Autodesk Fusion 360 part; units mm, degrees
(part 2 of 2)
  constraint tangent L247 A253
  constraint tangent L251 A253
  constraint concentric A111 A254
  constraint concentric A112 A255
  constraint tangent L109 A256
  constraint tangent L109 A257
  constraint tangent A258 L252
  constraint tangent L108 A259
  constraint tangent L252 A259
  constraint tangent L108 A260
  constraint tangent L199 A261
  constraint tangent L200 A261
  constraint tangent L192 A262
  constraint tangent L193 A262
  constraint tangent L174 A263
  constraint tangent L190 A263
  constraint tangent L183 A264
  constraint tangent L184 A264
  measures "d1" diameter of A0
  measures "d2" diameter of A1
  measures "d3" diameter of A2
  measures "d4" diameter of A3
  measures "d5" diameter of A4
  measures "d9" diameter of A111
  measures "d12" diameter of A112
  measures "d305" diameter of A254
  measures "d306" diameter of A255
extrude "Extrude1" add sketch "mriya-bumper-sla" along normal blind 10.5 contours L106 L107 L211 A215 L212 L228 L229 A231 | L106 L107 L202 A206 L203 A207 L204 A208 L205 A209 L206 A210 L207 A211 L208 A212 L209 A213 L210 A214 L211 L212 A216 L213 A217 L214 A218 L215 A219 L216 A220 L217 A221 L218 A222 L219 A223 L220 A224 L221 A225 L222 A226 L223 A227 L224 L225 L226 L227 L228 L229 L230 L231 L232 L233 L234 L235 L236 L237 L238 L239 L240 L241 L242 L243 L244 L245 A228 A229 A230 A232 A233 A234 A235 A236 A237 A238 A239 A240 A241 A242 A243 A244 A245 A246 A247 A248 A249 makes body 1
extrude "Extrude2" add sketch "mriya-bumper-sla" along normal blind 17 contours L106 L107 L211 A215 L212 L228 L229 A231 bodies 1
extrude "Extrude3" add sketch "mriya-bumper-sla" along normal blind 2 from surface at 1.7 contours L108 L109 L202 A206 L203 A207 L204 A208 L205 A209 L206 A210 L207 A211 L208 A212 L209 A213 L210 A214 L211 L212 A216 L213 A217 L214 A218 L215 A219 L216 A220 L217 A221 L218 A222 L219 A223 L220 A224 L221 A225 L222 A226 L223 A227 A256 A257 A258 L252 A259 A260 | L109 L212 A256 A257 | L108 L211 A215 L212 A258 L252 A259 A260 | A114 | A115 | A116 | A117 | A254 | A255 bodies 1
extrude "Extrude6" add sketch "mriya-bumper-sla" along normal blind 1 from surface at 14.3 contours L108 L211 A215 L212 A258 L252 A259 A260 bodies 1
extrude "Extrude14" add sketch "mriya-bumper-sla" along normal blind 1 from surface at 7.7 contours L109 L212 A256 A257 bodies 1
chamfer "Chamfer5" distance 0.599 angle 45 4 edges at (-14.85, 78.0932, 14.3) (-7.4686, 77.6246, 14.3) (-7, 58.2443, 14.3) (-7, 9.5932, 7.7) on bodies 1
sketch "power-switch" plane through (-4.5, 0, 0) normal (1, 0, 0) x (0, 1, 0)
  line L0 (1.9932, 0) -> (76.4932, 0)
  line L1 (76.4932, 0) -> (76.4932, 17)
  line L2 (76.4932, 17) -> (19.2932, 17)
  line L3 (19.2932, 17) -> (19.2932, 10.5)
  line L4 (19.2932, 10.5) -> (1.9932, 10.5)
  line L5 (1.9932, 10.5) -> (1.9932, 0)
  line L6 (36.0432, 5.4) -> (25.7432, 5.4)
  line L7 (25.7432, 5.4) -> (25.7432, 8.2)
  line L8 (25.7432, 8.2) -> (36.0432, 8.2)
  line L9 (36.0432, 8.2) -> (36.0432, 5.4)
  line L10 (36.6432, 3.8) -> (25.1432, 3.8)
  line L11 (24.1432, 4.8) -> (24.1432, 8.8)
  line L12 (25.1432, 9.8) -> (36.6432, 9.8)
  line L13 (37.6432, 8.8) -> (37.6432, 4.8)
  arc A0 (25.1432, 9.8) -> (24.1432, 8.8) centre (25.1432, 8.8) ccw
  arc A1 (37.6432, 8.8) -> (36.6432, 9.8) centre (36.6432, 8.8) ccw
  arc A2 (36.6432, 3.8) -> (37.6432, 4.8) centre (36.6432, 4.8) ccw
  arc A3 (24.1432, 4.8) -> (25.1432, 3.8) centre (25.1432, 4.8) ccw
  line L14 (19.2932, 10.5) -> (1.8932, 10.5)
  line L15 (1.8932, 10.5) -> (1.8932, 0)
  line L16 (1.8932, 0) -> (76.5932, 0)
  line L17 (76.5932, 0) -> (76.5932, 17)
  line L18 (76.5932, 17) -> (19.2932, 17)
  line L19 (19.2932, 17) -> (19.2932, 10.5)
  constraint perpendicular L6 L7
  constraint tangent L11 A0
  constraint tangent L12 A0
  constraint tangent L12 A1
  constraint tangent L13 A1
  constraint tangent L10 A2
  constraint tangent L13 A2
  constraint tangent L10 A3
  constraint tangent L11 A3
  constraint vertical L7
  constraint perpendicular L7 L8
  constraint vertical L9
extrude "Extrude8" cut sketch "power-switch" against normal blind 2.5 contours L6 L7 L8 L9 bodies 1
extrude "Extrude9" cut sketch "power-switch" against normal blind 1 contours L10 L11 L12 L13 A0 A1 A2 A3 bodies 1
chamfer "Chamfer4" distance 0.5 angle 45 4 edges at (-7, 30.8932, 5.4) (-7, 36.0432, 6.8) (-7, 30.8932, 8.2) (-7, 25.7432, 6.8) on bodies 1
sketch "usb-c" plane through (0, 80.5932, 0) normal (0, 1, 0) x (-1, 0, 0)
  line L0 (8.5, 0) -> (41.1088, 0)
  line L1 (41.1088, 0) -> (41.1088, 10.5)
  line L2 (41.1088, 10.5) -> (25.8, 10.5)
  line L3 (25.8, 10.5) -> (25.8, 17)
  line L4 (25.8, 17) -> (8.5, 17)
  line L5 (8.5, 17) -> (8.5, 0)
  line L6 (10.9002, 11.05) -> (10.9002, 10.15)
  arc A0 (21.0002, 11.05) -> (19.7002, 12.35) centre (19.7002, 11.05) ccw
  arc A1 (11.8003, 10.15) -> (13.1003, 8.85) centre (13.1002, 10.15) ccw
  line L7 (21.9002, 11.05) -> (21.9002, 10.15)
  line L8 (13.1002, 12.35) -> (19.7002, 12.35)
  line L9 (11.8003, 10.15) -> (11.8003, 11.05)
  line L10 (13.1002, 13.25) -> (19.7002, 13.25)
  line L11 (19.7002, 7.95) -> (13.1002, 7.95)
  arc A2 (13.1002, 12.35) -> (11.8003, 11.05) centre (13.1002, 11.05) ccw
  line L12 (19.7002, 8.85) -> (13.1002, 8.85)
  line L13 (21.0002, 11.05) -> (21.0002, 10.15)
  arc A3 (19.7002, 8.85) -> (21.0002, 10.15) centre (19.7003, 10.15) ccw
  arc A4 (13.1002, 13.25) -> (10.9002, 11.05) centre (13.1002, 11.05) ccw
  arc A5 (10.9002, 10.15) -> (13.1002, 7.95) centre (13.1002, 10.15) ccw
  arc A6 (21.9002, 11.05) -> (19.7003, 13.25) centre (19.7003, 11.05) ccw
  arc A7 (19.7002, 7.95) -> (21.9002, 10.15) centre (19.7002, 10.15) ccw
  constraint horizontal L11
  constraint tangent L9 A2
  constraint tangent L8 A2
  constraint tangent A1 L12
  constraint tangent A1 L9
  constraint tangent A0 L8
  constraint tangent A0 L13
  constraint tangent L13 A3
  constraint tangent L12 A3
  constraint parallel L7 L9
  constraint tangent L6 A4
  constraint tangent L10 A4
  constraint tangent L11 A5
  constraint tangent L6 A5
  constraint tangent L10 A6
  constraint tangent L7 A6
  constraint tangent L7 A7
  constraint tangent L11 A7
extrude "Extrude10" cut sketch "usb-c" against normal blind 2.5 contours A0 A1 L8 L9 A2 L12 L13 A3 bodies 1
extrude "Extrude11" cut sketch "usb-c" against normal blind 1 contours L6 L7 L10 L11 A4 A5 A6 A7 bodies 1
fillet "Fillet30" radius 0.5 4 edges at (-5.75, 19.2932, 10.5) (-5.75, 19.2932, 17) (-25.8, 79.3432, 10.5) (-25.8, 79.3432, 17) on bodies 1
fillet "Fillet27" radius 1.2 90 edges at (-4.5, 47.9432, 17) (-5.6716, 79.4216, 17) (-17.15, 80.5932, 17) (-33.4544, 80.5932, 10.5) (-41.4915, 80.6693, 10.5) (-42.3069, 81.3771, 10.5) (-43.9334, 82.6268, 10.5) (-51.5908, 82.8932, 10.5) (-58.2915, 82.9693, 10.5) (-60.2069, 84.7771, 10.5) (-62.9334, 87.1268, 10.5) (-73.4, 87.3932, 10.5) (-83.8666, 87.1268, 10.5) (-86.0931, 85.2771, 10.5) (-87.5085, 83.9693, 10.5) (-94.7092, 83.8932, 10.5) (-102.8666, 83.6268, 10.5) (-107.2698, 79.6003, 10.5) (-111.0243, 76.0074, 10.5) (-116.0627, 75.8932, 10.5) (-121.8666, 75.6268, 10.5) (-123.4931, 74.3771, 10.5) (-124.3085, 73.6693, 10.5) (-131.4456, 73.5932, 10.5) (-141.0284, 72.4216, 10.5) (-142.2, 42.8932, 10.5) (-141.0284, 13.3648, 10.5) (-120.4435, 12.1932, 10.5) (-100.9649, 12.5357, 10.5) (-96.4569, 16.5593, 10.5) (-92.76, 20.041, 10.5) (-84.5813, 20.1932, 10.5) (-75.6559, 19.7842, 10.5) (-70.5608, 11.5973, 10.5) (-65.0991, 3.0385, 10.5) (-55.8871, 2.4932, 10.5) (-48.3085, 2.4171, 10.5) (-47.4931, 1.7093, 10.5) (-45.8666, 0.4596, 10.5) (-37.1092, 0.1932, 10.5) (-29.3085, 0.1171, 10.5) (-28.4931, -0.5907, 10.5) (-26.8666, -1.8404, 10.5) (-17.0136, -2.1068, 10.5) (-5.6716, -0.9352, 10.5) (-4.5, 10.5932, 10.5) (-24.8044, 80.5932, 0) (-41.4915, 80.6693, 0) (-42.3069, 81.3771, 0) (-43.9334, 82.6268, 0) (-51.5908, 82.8932, 0) (-58.2915, 82.9693, 0) (-60.2069, 84.7771, 0) (-62.9334, 87.1268, 0) (-73.4, 87.3932, 0) (-83.8666, 87.1268, 0) (-86.0931, 85.2771, 0) (-87.5085, 83.9693, 0) (-94.7092, 83.8932, 0) (-102.8666, 83.6268, 0) (-107.2698, 79.6003, 0) (-111.0243, 76.0074, 0) (-116.0627, 75.8932, 0) (-121.8666, 75.6268, 0) (-123.4931, 74.3771, 0) (-124.3085, 73.6693, 0) (-131.4456, 73.5932, 0) (-141.0284, 72.4216, 0) (-142.2, 42.8932, 0) (-141.0284, 13.3648, 0) (-120.4435, 12.1932, 0) (-100.9649, 12.5357, 0) (-96.4569, 16.5593, 0) (-92.76, 20.041, 0) (-84.5813, 20.1932, 0) (-75.6559, 19.7842, 0) (-70.5608, 11.5973, 0) (-65.0991, 3.0385, 0) (-55.8871, 2.4932, 0) (-48.3085, 2.4171, 0) (-47.4931, 1.7093, 0) (-45.8666, 0.4596, 0) (-37.1092, 0.1932, 0) (-29.3085, 0.1171, 0) (-28.4931, -0.5907, 0) (-26.8666, -1.8404, 0) (-17.0136, -2.1068, 0) (-5.6716, -0.9352, 0) (-4.5, 39.2432, 0) (-5.6716, 79.4216, 0) on bodies 1
extrude "Extrude12" cut sketch "mriya-bumper-sla" along normal blind 1 from surface at 1.7 contours A254 | A255 bodies 1
chamfer "Chamfer6" distance 1 angle 45 8 edges at (-4.5, 30.8932, 9.8) (-4.5, 37.3503, 9.5071) (-4.5, 37.6432, 6.8) (-4.5, 37.3503, 4.0929) (-4.5, 30.8932, 3.8) (-4.5, 24.4361, 4.0929) (-4.5, 24.1432, 6.8) (-4.5, 24.4361, 9.5071) on bodies 1
chamfer "Chamfer7" distance 1 angle 45 8 edges at (-21.9003, 80.5932, 10.6) (-21.2559, 80.5932, 8.5944) (-16.4003, 80.5932, 7.95) (-11.5446, 80.5932, 8.5944) (-10.9003, 80.5932, 10.6) (-11.5446, 80.5932, 12.6056) (-16.4003, 80.5932, 13.25) (-21.2559, 80.5932, 12.6056) on bodies 1
mirror "Mirror1" about plane through (0, 0, 0) normal (1, 0, 0) of bodies 1 makes body 2
named bodies: "Left", "Right"
